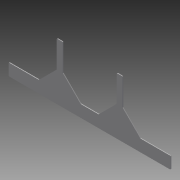
# Autodesk Inventor part: Strength Plate (0.125 Steel)
Saved by Autodesk Inventor 2014 (Build 180170000, 170)
## iProperties
Created: 2014-02-09
Part Number: Strength Plate (0.125 Steel)
Material: Steel
Document SubType Name: Modeling
Designer: Andrew Toennies
Mass: 1402.58 g
Surface Area: 1190.61 cm^2
Volume: 178.672 cm^3
Density: 7.85 g/cm^3
Appearance: Steel
Author: Andrew Toennies
Autodesk Inventor part; units mm, degrees
ref_plane "YZ Plane" through (0, 0, 0) normal (1, 0, 0) x (0, 1, 0)
ref_plane "XZ Plane" through (0, 0, 0) normal (0, 1, 0) x (-1, 0, 0)
ref_plane "XY Plane" through (0, 0, 0) normal (0, 0, 1) x (1, 0, 0)
sketch "Sketch1" plane through (0, 0, 0) normal (0, 0, 1) x (1, 0, 0)
  line L0 (3.175, 0) -> (685.8, 0)
  line L1 (688.975, 3.175) -> (688.975, 47.625)
  line L2 (0, 47.625) -> (0, 3.175)
  line L3 (204.7875, 128.3151) -> (204.7875, 238.125)
  line L4 (207.9625, 241.3) -> (227.0125, 241.3)
  line L5 (230.1875, 238.125) -> (230.1875, 128.3151)
  line L6 (458.7875, 128.3151) -> (458.7875, 238.125)
  line L7 (461.9625, 241.3) -> (481.0125, 241.3)
  line L8 (484.1875, 238.125) -> (484.1875, 128.3151)
  line L9 (203.8576, 126.0701) -> (129.5174, 51.7299)
  line L10 (231.1174, 126.0701) -> (305.4576, 51.7299)
  line L11 (457.8576, 126.0701) -> (383.5174, 51.7299)
  line L12 (485.1174, 126.0701) -> (559.4576, 51.7299)
  line L13 (127.2724, 50.8) -> (3.175, 50.8)
  line L14 (685.8, 50.8) -> (561.7026, 50.8)
  line L15 (381.2724, 50.8) -> (307.7026, 50.8)
  arc A0 (207.9625, 241.3) -> (204.7875, 238.125) centre (207.9625, 238.125) ccw
  arc A1 (230.1875, 238.125) -> (227.0125, 241.3) centre (227.0125, 238.125) ccw
  arc A2 (203.8576, 126.0701) -> (204.7875, 128.3151) centre (201.6125, 128.3151) ccw
  arc A3 (230.1875, 128.3151) -> (231.1174, 126.0701) centre (233.3625, 128.3151) ccw
  arc A4 (305.4576, 51.7299) -> (307.7026, 50.8) centre (307.7026, 53.975) ccw
  arc A5 (381.2724, 50.8) -> (383.5174, 51.7299) centre (381.2724, 53.975) ccw
  arc A6 (457.8576, 126.0701) -> (458.7875, 128.3151) centre (455.6125, 128.3151) ccw
  arc A7 (461.9625, 241.3) -> (458.7875, 238.125) centre (461.9625, 238.125) ccw
  arc A8 (484.1875, 238.125) -> (481.0125, 241.3) centre (481.0125, 238.125) ccw
  arc A9 (484.1875, 128.3151) -> (485.1174, 126.0701) centre (487.3625, 128.3151) ccw
  arc A10 (3.175, 50.8) -> (0, 47.625) centre (3.175, 47.625) ccw
  arc A11 (127.2724, 50.8) -> (129.5174, 51.7299) centre (127.2724, 53.975) ccw
  arc A12 (0, 3.175) -> (3.175, 0) centre (3.175, 3.175) ccw
  arc A13 (685.8, 0) -> (688.975, 3.175) centre (685.8, 3.175) ccw
  arc A14 (688.975, 47.625) -> (685.8, 50.8) centre (685.8, 47.625) ccw
  arc A15 (559.4576, 51.7299) -> (561.7026, 50.8) centre (561.7026, 53.975) ccw
  point P0 (0, 0)
  point P1 (688.975, 0)
  point P2 (688.975, 50.8)
  point P3 (128.5875, 50.8)
  point P4 (204.7875, 241.3)
  point P5 (230.1875, 241.3)
  point P6 (230.1875, 127)
  point P7 (458.7875, 241.3)
  point P8 (484.1875, 241.3)
  point P9 (484.1875, 127)
  point P10 (204.7875, 127)
  point P11 (306.3875, 50.8)
  point P12 (458.7875, 127)
  point P13 (560.3875, 50.8)
  dimension "d0" = 688.975
  dimension "d1" = 50.8
  dimension "d3" = 25.4
  dimension "d5" = 25.4
  dimension "d6" = 204.7875
  dimension "d7" = 204.7875
  dimension "d14" = 135
  dimension "d15" = 135
  dimension "d16" = 76.2
  dimension "d17" = 76.2
  dimension "d18" = 190.5
  dimension "d19" = 76.2
  dimension "d20" = 76.2
  dimension "d21" = 3.175
  constraints: 32 end point, 32 point on circle, 32 tangent, 28 point on line, 16 centre point, 15 equal radius, 11 perpendicular, 6 parallel, 3 collinear, 1 horizontal
  measures "d0" distance of point (0, 0) point (688.975, 0)
  measures "d1" distance of point (688.975, 0) point (688.975, 50.8)
  measures "d3" distance of point (204.787, 241.3) point (230.187, 241.3)
  measures "d5" distance of point (458.787, 241.3) point (484.187, 241.3)
  measures "d6" distance between parallel lines of L1 L8
  measures "d7" distance between parallel lines of L2 L3
  measures "d14" angle of L11 L15
  measures "d15" angle of L14 L12
  measures "d16" horizontal distance of point (204.788, 127) point (128.588, 50.8)
  measures "d17" horizontal distance of point (306.387, 50.8) point (230.187, 127)
  measures "d18" distance between parallel lines of L15 L4
  measures "d19" distance from line of L15 point (458.787, 127)
  measures "d20" horizontal distance of point (560.388, 50.8) point (484.188, 127)
  measures "d21" radius of A0
extrude "Extrusion1" add sketch "Sketch1" along normal blind 3.175
body "Solid1"
